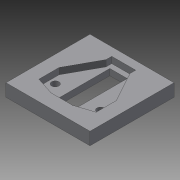
# Autodesk Inventor part: InkjetHolder
Saved by Autodesk Inventor 2015 (Build 190159000, 159)
## iProperties
Created: 2015-06-18
Part Number: InkjetHolder
Material: Generic
Document SubType Name: Modeling
Designer: Oliver
Density: 1 g/cm^3
Appearance: Default
Author: Oliver
Autodesk Inventor part; units mm, degrees
ref_plane "YZ Plane" through (0, 0, 0) normal (1, 0, 0) x (0, 1, 0)
ref_plane "XZ Plane" through (0, 0, 0) normal (0, 1, 0) x (-1, 0, 0)
ref_plane "XY Plane" through (0, 0, 0) normal (0, 0, 1) x (1, 0, 0)
sketch "Sketch1" plane through (0, 0, 0) normal (0, 0, 1) x (1, 0, 0)
  line L0 (-5, -2.5) -> (5, -2.5) construction
  line L1 (5, -2.5) -> (12.675, 0) construction
  line L2 (-5, -2.5) -> (-12.675, 0)
  line L3 (12.675, 0) -> (-12.675, 0) construction
  line L4 (12.675, 0) -> (12.675, 8.7) construction
  line L5 (-12.675, 0) -> (-12.675, 8.7)
  line L6 (-12.675, 8.7) -> (-4.75, 23.1)
  line L7 (-4.75, 23.1) -> (-4.75, 25.1)
  line L8 (-4.75, 25.1) -> (4.75, 25.1) construction
  line L9 (4.75, 25.1) -> (4.75, 23.1) construction
  line L10 (4.75, 23.1) -> (12.675, 8.7) construction
  line L11 (0, -9.3621) -> (0, 31.9621) projected
  line L12 (0, 25.1) -> (0, -2.5)
  circle A0 centre (-10.8, 4.25) radius 1.25
  line L13 (-10.8, 4.25) -> (0, 4.25) construction
  line L14 (-4.75, 25.1) -> (0, 25.1)
  line L15 (-5, -2.5) -> (0, -2.5)
  line L16 (-5.7087, 23.3464) -> (-13.6337, 8.9464)
  line L17 (-13.6337, 8.9464) -> (-13.6337, -0.696)
  line L18 (-13.6337, -0.696) -> (-5.1522, -3.4587)
  line L19 (-5.1522, -3.4587) -> (0.9587, -3.4587) construction
  line L20 (0.9587, -3.4587) -> (0.9587, 26.0587) construction
  line L21 (0.9587, 26.0587) -> (-5.7087, 26.0587) construction
  line L22 (-5.7087, 26.0587) -> (-5.7087, 23.3464)
  line L23 (0, -2.5) -> (0, -3.4587)
  line L24 (0, 25.1) -> (0, 26.0587)
  line L25 (0, -3.4587) -> (-5.1522, -3.4587)
  line L26 (0, 26.0587) -> (-5.7087, 26.0587)
  point P0 (0, 0)
  point P1 (0, 0)
  dimension "d0" = 10
  dimension "d1" = 25.35
  dimension "d2" = 2.5
  dimension "d3" = 8.7
  dimension "d4" = 27.6
  dimension "d6" = 2
  dimension "d7" = 9.5
  dimension "d42" = 2.5
  dimension "d43" = 10.8
  dimension "d44" = 6.75
  dimension "d53" = 0.9587
  constraints: 52 end point, 7 point on line, 4 equal length, 4 horizontal, 4 vertical, 3 collinear, 3 midpoint, 1 centre point, 1 coincident, 1 perpendicular, 6 other
  measures "d0" distance of L0.start L0.end
  measures "d1" distance of L1.end L2.end
  measures "d2" distance between parallel lines of L3 L0
  measures "d3" distance of L1.end L4.end
  measures "d4" distance between parallel lines of L0 L8
  measures "d6" distance of L8.end L9.end
  measures "d7" distance of L7.end L8.end
  measures "d42" diameter of A0
  measures "d43" distance of L13.start L13.end
  measures "d44" distance between parallel lines of L0 L13
  measures "d53" distance between parallel lines of L6 L16
sketch "Sketch8" plane through (0, 0, 0) normal (0, 0, 1) x (1, 0, 0)
  line L0 (-20, 30) -> (20, 30)
  line L1 (20, 30) -> (20, -10)
  line L2 (20, -10) -> (-20, -10)
  line L3 (-20, -10) -> (-20, 30)
  point P0 (0, 0)
  point P1 (0, -10)
  dimension "d45" = 40
  dimension "d46" = 10
  constraints: 8 end point, 2 parallel, 2 perpendicular, 1 horizontal, 1 midpoint, 1 vertical alignment
  measures "d45" distance of L1.end L2.end
  measures "d46" distance from line of L2 point (0, 0)
extrude "MainBlock" add sketch "Sketch8" against normal blind 6
extrude "CartridgeCutout" cut sketch "Sketch1" against normal blind 3
sketch "Sketch10" plane through (-10.8, 4.25, 0) normal (0, 0, 1) x (1, 0, 0)
  circle A0 centre (0, 0) radius 1.25 projected
  circle A1 centre (0, 0) radius 1.75
  point P0 (10.8, -4.25)
  dimension "d56" = 0.5
  constraints: 1 centre point
  measures "d56" radial gap between concentric circles of A0 A1
extrude "PinHole" cut sketch "Sketch10" against normal through all contours A0 | A1
mirror "Mirror3" about plane through (0, 26.0587, 0) normal (-1, 0, 0) of "CartridgeCutout", "PinHole"
sketch "Sketch12" plane through (0, 0, -3) normal (0, 0, 1) x (1, 0, 0)
  circle A0 centre (10.8, 4.25) radius 1.75 projected
  circle A1 centre (-10.8, 4.25) radius 1.75 projected
  line L0 (5.7087, 26.0587) -> (-5.7087, 26.0587) projected
  line L1 (-5.7087, 23.3464) -> (-5.7087, 26.0587) projected
  line L2 (-13.6337, 8.9464) -> (-5.7087, 23.3464) projected
  line L3 (-13.6337, -0.696) -> (-13.6337, 8.9464) projected
  line L4 (-5.1522, -3.4587) -> (-13.6337, -0.696) projected
  line L5 (5.1522, -3.4587) -> (-5.1522, -3.4587) projected
  line L6 (5.1522, -3.4587) -> (13.6337, -0.696) projected
  line L7 (13.6337, -0.696) -> (13.6337, 8.9464) projected
  line L8 (13.6337, 8.9464) -> (5.7087, 23.3464) projected
  line L9 (5.7087, 23.3464) -> (5.7087, 26.0587) projected
  line L10 (-4.15, 23.6) -> (4.15, 23.6)
  line L11 (4.15, 23.6) -> (4.15, -1.4)
  line L12 (4.15, -1.4) -> (-4.15, -1.4)
  line L13 (-4.15, -1.4) -> (-4.15, 23.6)
  point P0 (0, 0)
  point P1 (0, -1.4)
  dimension "d59" = 8.3
  dimension "d60" = 25
  dimension "d61" = 1.4
  constraints: 8 end point, 2 parallel, 1 horizontal, 1 midpoint, 1 perpendicular, 1 vertical alignment
  measures "d59" distance of L11.end L12.end
  measures "d60" distance of L10.end L11.end
  measures "d61" distance from line of L12 point (0, 0)
extrude "Extrusion12" cut sketch "Sketch12" against normal through all contours L10 L11 L12 L13
body "Solid4"
